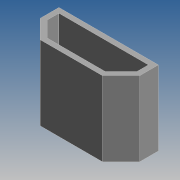
# Autodesk Inventor part: R005
Saved by Autodesk Inventor 2017 (Build 210142000, 142)
## iProperties
Created: 2018-10-19
Part Number: R005
Material: Acier / Stahl
Document SubType Name: Modeling
Designer: Gilles Mottiez
Density: 7.85 g/cm^3
Appearance: Par défaut
Description: Connecteur micro USB Raspberry pi 3B
Author: Gilles Mottiez
Autodesk Inventor part; units mm, degrees
ref_plane "YZ Plane" through (0, 0, 0) normal (1, 0, 0) x (0, 1, 0)
ref_plane "XZ Plane" through (0, 0, 0) normal (0, 1, 0) x (-1, 0, 0)
ref_plane "XY Plane" through (0, 0, 0) normal (0, 0, 1) x (1, 0, 0)
sketch "Sketch1" plane through (0, 0, 0) normal (0, 0, 1) x (1, 0, 0)
  line L0 (0, 0) -> (8, 0) construction
  line L1 (8, 0) -> (8, 3) construction
  line L2 (8, 3) -> (0, 3) construction
  line L3 (0, 3) -> (0, 0) construction
  line L4 (1.5, 0) -> (6.5, 0) construction
  line L5 (6.5, 0) -> (6.5, 3) construction
  line L6 (6.5, 3) -> (1.5, 3) construction
  line L7 (1.5, 3) -> (1.5, 0) construction
  line L8 (4, 3) -> (4, 0) construction
  line L9 (0, 3) -> (8, 3) construction
  line L10 (8, 3) -> (8, 1.5) construction
  line L11 (8, 1.5) -> (0, 1.5) construction
  line L12 (0, 1.5) -> (0, 3) construction
  line L13 (0, 3) -> (8, 3)
  line L14 (8, 3) -> (8, 1.5)
  line L15 (8, 1.5) -> (6.5, 0)
  line L16 (6.5, 0) -> (1.5, 0)
  line L17 (1.5, 0) -> (0, 1.5)
  line L18 (0, 1.5) -> (0, 3)
  line L19 (0.4, 1.6657) -> (1.6657, 0.4)
  line L20 (1.6657, 0.4) -> (6.3343, 0.4)
  line L21 (6.3343, 0.4) -> (7.6, 1.6657)
  line L22 (7.6, 1.6657) -> (7.6, 2.6)
  line L23 (7.6, 2.6) -> (0.4, 2.6)
  line L24 (0.4, 2.6) -> (0.4, 1.6657)
  dimension "d0" = 8
  dimension "d1" = 3
  dimension "d2" = 5
  dimension "d3" = 1.5
  dimension "d4" = 0.4
  constraints: 50 end point, 6 parallel, 4 perpendicular, 3 collinear, 3 horizontal, 3 midpoint, 2 point on line, 6 other
  measures "d0" distance of L2.end L1.end
  measures "d1" distance of L2.end L0.start
  measures "d2" distance of L6.end L5.end
  measures "d3" distance of L9.end L10.end
  measures "d4" distance between parallel lines of L17 L19
extrude "Extrusion1" add sketch "Sketch1" against normal blind 6
sketch "Esquisse2" plane through (0, 0, -6) normal (0, 0, -1) x (-1, 0, 0)
  line L0 (-6.5, 0) -> (-1.5, 0) projected
  line L1 (-8, 1.5) -> (-6.5, 0) projected
  line L2 (-8, 3) -> (-8, 1.5) projected
  line L3 (0, 3) -> (-8, 3) projected
  line L4 (0, 1.5) -> (0, 3) projected
  line L5 (-1.5, 0) -> (0, 1.5) projected
  point P0 (0, 0)
extrude "Extrusion2" add sketch "Esquisse2" against normal blind 1
